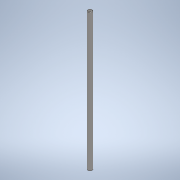
# Autodesk Inventor part: Z-Axis Rod
Saved by Autodesk Inventor 2020 (Build 240168000, 168)
## iProperties
Created: 2019-06-17
Part Number: Z-Axis Rod
Material: Stainless Steel, 440C
Document SubType Name: Modeling
Designer: pepd9
Density: 7.75 g/cm^3
Appearance: Semi-Polished
Author: pepd9
Autodesk Inventor part; units mm, degrees
ref_plane "YZ Plane" through (0, 0, 0) normal (1, 0, 0) x (0, 1, 0)
ref_plane "XZ Plane" through (0, 0, 0) normal (0, 1, 0) x (-1, 0, 0)
ref_plane "XY Plane" through (0, 0, 0) normal (0, 0, 1) x (1, 0, 0)
sketch "Sketch1" plane through (0, 0, 0) normal (0, 1, 0) x (-1, 0, 0)
  circle A0 centre (0, 0) radius 5
  dimension "d0" = 10
  constraints: 1 centre point, 1 coincident
  measures "d0" diameter of A0
extrude "Extrusion1" add sketch "Sketch1" along normal blind 320
chamfer "Chamfer1" distance 1 angle 45 2 edges at (5, 320, 0) (5, 0, 0)
body "Solid1"
